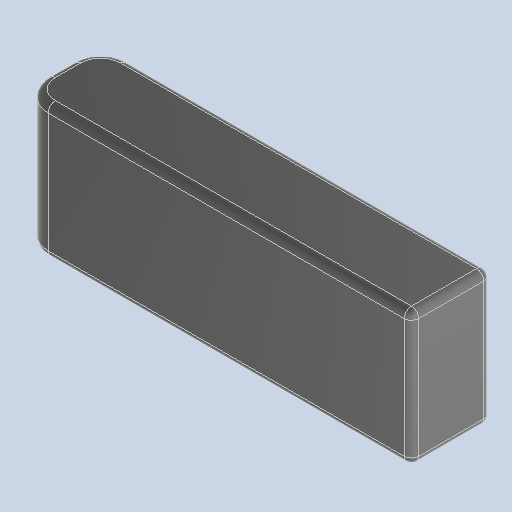
# Autodesk Inventor part: Lipo-2800-3S-Pack-3
Saved by Autodesk Inventor 2024.2 (Build 282272000, 272)
## iProperties
Created: 2024-01-26
Part Number: Lipo-2800-3S-Pack-3
Material: Acetal Resin, Black
Document SubType Name: Modeling
Designer: Masato Kubotera
Mass: 188 g
Surface Area: 135.826 cm^2
Volume: 86.5276 cm^3
Density: 2.17272 g/cm^3
Appearance: Smooth - Black
Catalog Web Link: https://maxamps.com/products/lipo-2800-3s-11-1v-battery-pack
Vendor: MaxAmps
Author: Masato Kubotera
Autodesk Inventor part; units mm, degrees
ref_plane "YZ Plane" through (0, 0, 0) normal (1, 0, 0) x (0, 1, 0)
ref_plane "XZ Plane" through (0, 0, 0) normal (0, 1, 0) x (-1, 0, 0)
ref_plane "XY Plane" through (0, 0, 0) normal (0, 0, 1) x (1, 0, 0)
sketch "Sketch1" plane through (0, 0, 0) normal (0, 0, 1) x (1, 0, 0)
  line L0 (-11, -54) -> (11, -54)
  line L1 (11, -54) -> (11, 54)
  line L2 (11, 54) -> (-11, 54)
  line L3 (-11, 54) -> (-11, -54)
  line L4 (-11, -54) -> (11, 54) construction
  line L5 (11, -54) -> (-11, 54) construction
  point P0 (0, 0)
  dimension "d0" = 22
  dimension "d1" = 108
  constraints: 12 end point, 2 midpoint, 2 parallel, 1 horizontal, 1 perpendicular
  measures "d0" distance of L1.end L2.end
  measures "d1" distance of L0.end L1.end
extrude "Extrusion1" add sketch "Sketch1" along normal blind 37
fillet "Fillet1" radius 2 10 edges at (11, 54, 18.5) (-11, 54, 18.5) (0, 54, 37) (11, 0, 37) (-11, 0, 37) (11, 0, 0) (0, 54, 0) (-11, 0, 0) (0, -54, 37) (0, -54, 0)
fillet "Fillet2" radius 7.5 6 edges at (10.4142, -53.4142, 36.4142) (10.4142, -53.4142, 0.5858) (11, -54, 18.5) (-10.4142, -53.4142, 36.4142) (-10.4142, -53.4142, 0.5858) (-11, -54, 18.5)
body "Solid1"
